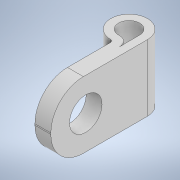
# Autodesk Inventor part: Cable Clip 3-1Dia RS817-8956
Saved by Autodesk Inventor 2021 (Build 250183000, 183)
## iProperties
Created: 2020-08-05
Part Number: Cable Clip 3-1Dia RS817-8956
Material: Generic
Document SubType Name: Modeling
Designer: jgray
Density: 1 g/cm^3
Appearance: Default
Author: jgray
Autodesk Inventor part; units mm, degrees
ref_plane "YZ Plane" through (0, 0, 0) normal (1, 0, 0) x (0, 1, 0)
ref_plane "XZ Plane" through (0, 0, 0) normal (0, 1, 0) x (-1, 0, 0)
ref_plane "XY Plane" through (0, 0, 0) normal (0, 0, 1) x (1, 0, 0)
sketch "Sketch1" plane through (0, 0, 0) normal (0, 1, 0) x (-1, 0, 0)
  arc A0 (-1.55, 0) -> (-0.0788, 1.548) centre (0, 0) ccw
  line L0 (-1.55, 14.25) -> (-1.55, 0)
  arc A1 (-1.55, 2.9462) -> (-0.0788, 1.548) centre (-0.15, 2.9462) ccw
  arc A2 (-0.35, 3.0996) -> (0.0435, 2.6996) centre (0.05, 3.0996) ccw
  line L1 (-1.55, 14.25) -> (-0.35, 14.25)
  line L2 (-0.35, 14.25) -> (-0.35, 3.0996)
  line L3 (-2.7, 14.25) -> (-2.7, 0)
  line L4 (-2.7, 14.25) -> (-1.55, 14.25)
  arc A3 (-2.7, 0) -> (0.0435, 2.6996) centre (0, 0) ccw
  dimension "d0" = 3.1
  dimension "d1" = 2.8
  dimension "d2" = 14.25
  dimension "d6" = 0.8
  constraints: 10 end point, 8 point on circle, 5 tangent, 4 centre point, 3 vertical, 2 coincident, 1 horizontal, 1 perpendicular, 1 point on line
  measures "d0" diameter of A0
  measures "d1" diameter of A1
  measures "d2" vertical distance of point (0, 0) L0.start
  measures "d6" diameter of A2
extrude "Extrusion1" add sketch "Sketch1" along normal blind 9.8
sketch "Sketch2" plane through (0.35, 0, 3.0996) normal (-1, 0, 0) x (0, 0, 1)
  line L0 (6.0004, -8.6055) -> (6.0004, 17.2383) construction
  line L1 (-11.7051, 4.9) -> (18.5644, 4.9) construction
  line L2 (11.1504, 0) -> (11.1504, 9.8) construction
  line L3 (-3.0996, 0) -> (-0.3999, 0) construction
  line L4 (-0.3999, 0) -> (-0.3999, 9.8) construction
  line L5 (-3.0996, 9.8) -> (-0.3999, 9.8) construction
  line L6 (-3.0996, 0) -> (-3.0996, 9.8) construction
  line L7 (-3.0996, 0) -> (-3.0996, 9.8) construction
  line L8 (-5.7996, 0) -> (-5.7996, 9.8) construction
  point P0 (11.1504, 4.9)
  point P1 (6.0004, 4.9)
  dimension "d9" = 11.8
  constraints: 4 end point, 3 point on line, 1 horizontal, 1 midpoint, 1 vertical
  measures "d9" distance between parallel lines of L0 L8
hole "Hole1" at (0.35, 4.9, 9.1) direction (1, 0, 0) diameter 4.8 end through all
fillet "Fillet1" radius 4.8 2 edges at (1.525, 9.8, 14.25) (1.525, 0, 14.25)
body "Solid1"
